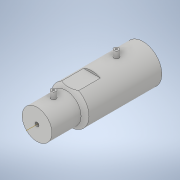
# Autodesk Inventor part: int 3.2
Saved by Autodesk Inventor 2020 (Build 240168000, 168)
## iProperties
Created: 2019-10-25
Part Number: int 3.2
Material: Genérico
Document SubType Name: Modeling
Designer: Camila Angel
Density: 1 g/cm^3
Appearance: Valor por defecto
Author: Camila Angel
Autodesk Inventor part; units mm, degrees
sketch "Boceto1" plane through (0, 0, 0) normal (0, 0, 1) x (1, 0, 0)
  circle A0 centre (0, 0) radius 11.25
  circle A1 centre (0, 0) radius 14.25
  dimension "d0" = 22.5
  dimension "d1" = 3
  constraints: 2 centre point, 1 coincident
  measures "d0" diameter of A0
  measures "d1" radial gap between concentric circles of A0 A1
extrude "Extrusión1" add sketch "Boceto1" along normal blind 55
sketch "Boceto2" plane through (0, 0, 55) normal (0, 0, 1) x (1, 0, 0)
  circle A0 centre (0, 0) radius 11.25
  circle A1 centre (0, 0) radius 1.5
  dimension "d4" = 22.5
  dimension "d5" = 3
  constraints: 2 centre point, 2 coincident
  measures "d4" diameter of A0
  measures "d5" diameter of A1
extrude "Extrusión2" add sketch "Boceto2" along normal blind 25 and the other way blind 15
chamfer "Chaflán1" distance 3 angle 45 1 edges at (-11.25, 0, 55)
sketch "Boceto5" plane through (0, 0, 0) normal (1, 0, 0) x (0, 1, 0)
  line L0 (11.25, 58) -> (11.25, 80) construction
  line L1 (14.25, 0) -> (14.25, 55) construction
  point P0 (0, 0)
ref_plane "Plano de trabajo1" through (0, 11.25, 58) normal (0, 1, 0) x (-1, 0, 0)
sketch "Boceto6" plane through (0, 11.25, 58) normal (0, 1, 0) x (-1, 0, 0)
  circle A0 centre (0, 9.5303) radius 1.5
  circle A1 centre (0, 9.5303) radius 0.75
  point P0 (0, -58)
  dimension "d21" = 3
  dimension "d22" = 0.75
  constraints: 2 centre point
  measures "d21" diameter of A0
  measures "d22" radial gap between concentric circles of A0 A1
extrude "Extrusión4" add sketch "Boceto6" along normal blind 5
extrude "Extrusión5" add sketch "Boceto6" against normal up to next
ref_plane "Plano de trabajo2" through (0, 14.25, 0) normal (0, 1, 0) x (-1, 0, 0)
sketch "Boceto7" plane through (0, 14.25, 0) normal (0, 1, 0) x (-1, 0, 0)
  circle A0 centre (0, 20) radius 1.5
  circle A1 centre (0, 20) radius 0.75
  line L0 (-14.25, 0) -> (14.25, 0) projected
  point P0 (0, 0)
  dimension "d27" = 3
  dimension "d28" = 1.5
  dimension "d29" = 20
  constraints: 2 centre point, 1 coincident
  measures "d27" diameter of A0
  measures "d28" diameter of A1
  measures "d29" distance from line of A0.centre L0
extrude "Extrusión6" add sketch "Boceto7" along normal blind 5
extrude "Extrusión7" add sketch "Boceto7" against normal up to next
extrude "Extrusión8" cut sketch "Boceto6" against normal blind 10 contours A1
extrude "Extrusión9" cut sketch "Boceto7" against normal blind 10 contours A1
fillet "Empalme1" radius 8.25 1 edges at (-11.25, 0, 40)
sketch "Boceto9" plane through (0, 0, 80) normal (0, 0, 1) x (1, 0, 0)
  circle A0 centre (0, 0) radius 11.25 construction
  line L0 (-11.25, 0) -> (11.25, 0) construction
  constraints: 2 end point, 2 point on circle, 1 horizontal
ref_plane "Plano de trabajo3" through (-14.25, 0, 0) normal (1, 0, 0) x (0, 1, 0)
sketch "Boceto10" plane through (-14.25, 0, 0) normal (1, 0, 0) x (0, 1, 0)
  line L0 (14.25, 0) -> (14.25, 55) construction
  line L1 (11.25, 58) -> (14.25, 55) construction
  line L2 (11.25, 58) -> (11.25, 80) construction
  line L3 (12.75, 56.5) -> (14.25, 56.5)
  line L4 (14.25, 56.5) -> (14.25, 38.5)
  line L5 (14.25, 38.5) -> (12.75, 38.5)
  line L6 (12.75, 38.5) -> (12.75, 56.5)
  point P0 (0, 0)
  dimension "d53" = 1.5
  dimension "d54" = 18
  constraints: 8 end point, 2 parallel, 1 horizontal, 1 midpoint, 1 perpendicular, 1 point on line
  measures "d53" distance between parallel lines of L6 L0
  measures "d54" distance between parallel lines of L5 L3
extrude "Extrusión11" cut sketch "Boceto10" along normal blind 30
sketch "Boceto11" plane through (0, 0, 0) normal (1, 0, 0) x (0, 1, 0)
  line L0 (3, 40) -> (-3, 40) construction
  line L1 (-11.25, 31.75) -> (11.25, 31.75) construction
  line L2 (1.5, 40) -> (1.5, 80) construction
  arc A0 (11.25, 31.75) -> (3, 40) centre (3, 31.75) ccw construction
  line L3 (10.1447, 35.875) -> (1.5, 35.875)
  line L4 (1.5, 35.875) -> (1.5, 50.875)
  line L5 (10.1447, 35.875) -> (1.5, 50.875)
  line L6 (0, -16) -> (0, 96) projected
  point P0 (0, 0)
  dimension "d57" = 4.125
  dimension "d58" = 15
  constraints: 6 end point, 1 horizontal, 1 perpendicular, 1 point on circle, 1 point on line
  measures "d57" distance between parallel lines of L1 L3
  measures "d58" distance of L3.end L4.end
revolve "Revolución1" cut sketch "Boceto11" angle 360 about axis through (0, 0, -10) along (0, 0, 1)
sketch "Sketch12" plane through (0, 16.25, 67.5303) normal (0, 1, 0) x (1, 0, 0)
  circle A0 centre (0, 0) radius 1.9
  circle A1 centre (0, 0) radius 0.75 projected
  circle A2 centre (0, 0) radius 1.5 projected
  point P0 (0, 67.5303)
  dimension "d60" = 3.8
  constraints: 1 centre point
  measures "d60" diameter of A0
extrude "Extrusion12" add sketch "Sketch12" against normal up to surface contours A0 round surface about axis through (0, 0, 55) along (0, 0, 1) radius 11.25 far side no
sketch "Sketch13" plane through (0, 19.25, 20) normal (0, 1, 0) x (1, 0, 0)
  circle A0 centre (0, 0) radius 1.9
  circle A1 centre (0, 0) radius 0.75 projected
  circle A2 centre (0, 0) radius 1.5 projected
  point P0 (0, 20)
  dimension "d63" = 3.8
  constraints: 1 centre point
  measures "d63" diameter of A0
extrude "Extrusion13" add sketch "Sketch13" against normal up to surface contours A0 round surface about axis through (0, 0, 0) along (0, 0, 1) radius 14.25 far side no
